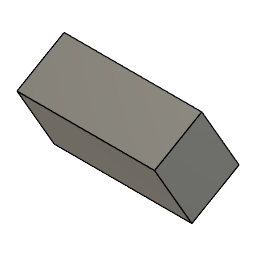
box_rx30_run01 (Autodesk Fusion 360 design; units mm, degrees)
Autodesk Fusion 360 part; units mm, degrees
ref_plane "工作平面1" through (12.125, 0, 0) normal (0, -0.5, 0.866025) x (1, 0, 0)
sketch "草图1" plane through (0, 0, 0) normal (0, -0.5, 0.866025) x (1, 0, 0)
  line L0 (0, 0) -> (48, 0)
  line L1 (48, 0) -> (48, 26)
  line L2 (48, 26) -> (0, 26)
  line L3 (0, 26) -> (0, 0)
extrude "拉伸1" add sketch "草图1" along normal blind 19
